Autodesk Fusion 360 part; units mm, degrees
(part 4 of 6)
sketch "b back lines" plane through (0, 0, 0) normal (0, 0, 1) x (1, 0, 0) in component "b back component"
  line L0 (155.185, 125.185) -> (161.93, 125.185)
  line L1 (161.93, 125.185) -> (161.93, 122.01)
  line L2 (161.93, 122.01) -> (172.09, 122.01)
  line L3 (172.09, 122.01) -> (172.09, 125.185)
  line L4 (172.09, 125.185) -> (181.93, 125.185)
  line L5 (181.93, 125.185) -> (181.93, 122.01)
  line L6 (181.93, 122.01) -> (192.09, 122.01)
  line L7 (192.09, 122.01) -> (192.09, 125.185)
  line L8 (192.09, 125.185) -> (201.93, 125.185)
  line L9 (201.93, 125.185) -> (201.93, 122.01)
  line L10 (201.93, 122.01) -> (212.09, 122.01)
  line L11 (212.09, 122.01) -> (212.09, 125.185)
  line L12 (212.09, 125.185) -> (221.93, 125.185)
  line L13 (221.93, 125.185) -> (221.93, 122.01)
  line L14 (221.93, 122.01) -> (232.09, 122.01)
  line L15 (232.09, 122.01) -> (232.09, 125.185)
  line L16 (232.09, 125.185) -> (241.93, 125.185)
  line L17 (241.93, 125.185) -> (241.93, 122.01)
  line L18 (241.93, 122.01) -> (252.09, 122.01)
  line L19 (252.09, 122.01) -> (252.09, 125.185)
  line L20 (252.09, 125.185) -> (261.93, 125.185)
  line L21 (261.93, 125.185) -> (261.93, 122.01)
  line L22 (261.93, 122.01) -> (272.09, 122.01)
  line L23 (272.09, 122.01) -> (272.09, 125.185)
  line L24 (272.09, 125.185) -> (281.93, 125.185)
  line L25 (281.93, 125.185) -> (281.93, 122.01)
  line L26 (281.93, 122.01) -> (292.09, 122.01)
  line L27 (292.09, 122.01) -> (292.09, 125.185)
  line L28 (292.09, 125.185) -> (298.835, 125.185)
  line L29 (298.835, 125.185) -> (298.835, 139.43)
  line L30 (298.835, 139.43) -> (302.01, 139.43)
  line L31 (302.01, 139.43) -> (302.01, 149.59)
  line L32 (302.01, 149.59) -> (298.835, 149.59)
  line L33 (298.835, 149.59) -> (298.835, 159.43)
  line L34 (298.835, 159.43) -> (302.01, 159.43)
  line L35 (302.01, 159.43) -> (302.01, 169.59)
  line L36 (302.01, 169.59) -> (298.835, 169.59)
  line L37 (298.835, 169.59) -> (298.835, 183.835)
  line L38 (155.185, 183.835) -> (161.93, 183.835)
  line L39 (161.93, 183.835) -> (161.93, 187.01)
  line L40 (161.93, 187.01) -> (172.09, 187.01)
  line L41 (172.09, 187.01) -> (172.09, 183.835)
  line L42 (172.09, 183.835) -> (181.93, 183.835)
  line L43 (181.93, 183.835) -> (181.93, 187.01)
  line L44 (181.93, 187.01) -> (192.09, 187.01)
  line L45 (192.09, 187.01) -> (192.09, 183.835)
  line L46 (192.09, 183.835) -> (201.93, 183.835)
  line L47 (201.93, 183.835) -> (201.93, 187.01)
  line L48 (201.93, 187.01) -> (212.09, 187.01)
  line L49 (212.09, 187.01) -> (212.09, 183.835)
  line L50 (212.09, 183.835) -> (221.93, 183.835)
  line L51 (221.93, 183.835) -> (221.93, 187.01)
  line L52 (221.93, 187.01) -> (232.09, 187.01)
  line L53 (232.09, 187.01) -> (232.09, 183.835)
  line L54 (232.09, 183.835) -> (241.93, 183.835)
  line L55 (241.93, 183.835) -> (241.93, 187.01)
  line L56 (241.93, 187.01) -> (252.09, 187.01)
  line L57 (252.09, 187.01) -> (252.09, 183.835)
  line L58 (252.09, 183.835) -> (261.93, 183.835)
  line L59 (261.93, 183.835) -> (261.93, 187.01)
  line L60 (261.93, 187.01) -> (272.09, 187.01)
  line L61 (272.09, 187.01) -> (272.09, 183.835)
  line L62 (272.09, 183.835) -> (281.93, 183.835)
  line L63 (281.93, 183.835) -> (281.93, 187.01)
  line L64 (281.93, 187.01) -> (292.09, 187.01)
  line L65 (292.09, 187.01) -> (292.09, 183.835)
  line L66 (292.09, 183.835) -> (298.835, 183.835)
  line L67 (155.185, 125.185) -> (155.185, 139.43)
  line L68 (155.185, 139.43) -> (152.01, 139.43)
  line L69 (152.01, 139.43) -> (152.01, 149.59)
  line L70 (152.01, 149.59) -> (155.185, 149.59)
  line L71 (155.185, 149.59) -> (155.185, 159.43)
  line L72 (155.185, 159.43) -> (152.01, 159.43)
  line L73 (152.01, 159.43) -> (152.01, 169.59)
  line L74 (152.01, 169.59) -> (155.185, 169.59)
  line L75 (155.185, 169.59) -> (155.185, 183.835)
  dimension "d5610" = 6.745
  dimension "d5611" = 3.175
  dimension "d5612" = 10.16
  dimension "d5613" = 3.175
  dimension "d5614" = 9.84
  dimension "d5615" = 3.175
  dimension "d5616" = 10.16
  dimension "d5617" = 3.175
  dimension "d5618" = 9.84
  dimension "d5619" = 3.175
  dimension "d5620" = 10.16
  dimension "d5621" = 3.175
  dimension "d5622" = 9.84
  dimension "d5623" = 3.175
  dimension "d5624" = 10.16
  dimension "d5625" = 3.175
  dimension "d5626" = 9.84
  dimension "d5627" = 3.175
  dimension "d5628" = 10.16
  dimension "d5629" = 3.175
  dimension "d5630" = 9.84
  dimension "d5631" = 3.175
  dimension "d5632" = 10.16
  dimension "d5633" = 3.175
  dimension "d5634" = 9.84
  dimension "d5635" = 3.175
  dimension "d5636" = 10.16
  dimension "d5637" = 3.175
  dimension "d5638" = 6.745
  dimension "d5653" = 14.245
  dimension "d5654" = 3.175
  dimension "d5655" = 10.16
  dimension "d5656" = 3.175
  dimension "d5657" = 9.84
  dimension "d5658" = 3.175
  dimension "d5659" = 10.16
  dimension "d5660" = 3.175
  dimension "d5661" = 14.245
  dimension "d5666" = 6.745
  dimension "d5667" = 3.175
  dimension "d5668" = 10.16
  dimension "d5669" = 3.175
  dimension "d5670" = 9.84
  dimension "d5671" = 3.175
  dimension "d5672" = 10.16
  dimension "d5673" = 3.175
  dimension "d5674" = 9.84
  dimension "d5675" = 3.175
  dimension "d5676" = 10.16
  dimension "d5677" = 3.175
  dimension "d5678" = 9.84
  dimension "d5679" = 3.175
  dimension "d5680" = 10.16
  dimension "d5681" = 3.175
  dimension "d5682" = 9.84
  dimension "d5683" = 3.175
  dimension "d5684" = 10.16
  dimension "d5685" = 3.175
  dimension "d5686" = 9.84
  dimension "d5687" = 3.175
  dimension "d5688" = 10.16
  dimension "d5689" = 3.175
  dimension "d5690" = 9.84
  dimension "d5691" = 3.175
  dimension "d5692" = 10.16
  dimension "d5693" = 3.175
  dimension "d5694" = 6.745
  dimension "d5709" = 14.245
  dimension "d5710" = 3.175
  dimension "d5711" = 10.16
  dimension "d5712" = 3.175
  dimension "d5713" = 9.84
  dimension "d5714" = 3.175
  dimension "d5715" = 10.16
  dimension "d5716" = 3.175
  dimension "d5717" = 14.245
  constraint horizontal L0
  constraint vertical L1
  constraint horizontal L2
  constraint vertical L3
  constraint horizontal L4
  constraint vertical L5
  constraint horizontal L6
  constraint vertical L7
  constraint horizontal L8
  constraint vertical L9
  constraint horizontal L10
  constraint vertical L11
  constraint horizontal L12
  constraint vertical L13
  constraint horizontal L14
  constraint vertical L15
  constraint horizontal L16
  constraint vertical L17
  constraint horizontal L18
  constraint vertical L19
  constraint horizontal L20
  constraint vertical L21
  constraint horizontal L22
  constraint vertical L23
  constraint horizontal L24
  constraint vertical L25
  constraint horizontal L26
  constraint vertical L27
  constraint horizontal L28
  constraint vertical L29
  constraint horizontal L30
  constraint vertical L31
  constraint horizontal L32
  constraint vertical L33
  constraint horizontal L34
  constraint vertical L35
  constraint horizontal L36
  constraint vertical L37
  constraint horizontal L38
  constraint vertical L39
  constraint horizontal L40
  constraint vertical L41
  constraint horizontal L42
  constraint vertical L43
  constraint horizontal L44
  constraint vertical L45
  constraint horizontal L46
  constraint vertical L47
  constraint horizontal L48
  constraint vertical L49
  constraint horizontal L50
  constraint vertical L51
  constraint horizontal L52
  constraint vertical L53
  constraint horizontal L54
  constraint vertical L55
  constraint horizontal L56
  constraint vertical L57
  constraint horizontal L58
  constraint vertical L59
  constraint horizontal L60
  constraint vertical L61
  constraint horizontal L62
  constraint vertical L63
  constraint horizontal L64
  constraint vertical L65
  constraint horizontal L66
  constraint vertical L67
  constraint horizontal L68
  constraint vertical L69
  constraint horizontal L70
  constraint vertical L71
  constraint horizontal L72
  constraint vertical L73
  constraint horizontal L74
  constraint vertical L75
  measures "d5610" distance of L0.start L0.end
  measures "d5611" distance of L0.end L1.end
  measures "d5612" distance of L1.end L2.end
  measures "d5613" distance of L2.end L3.end
  measures "d5614" distance of L3.end L4.end
  measures "d5615" distance of L4.end L5.end
  measures "d5616" distance of L5.end L6.end
  measures "d5617" distance of L6.end L7.end
  measures "d5618" distance of L7.end L8.end
  measures "d5619" distance of L8.end L9.end
  measures "d5620" distance of L9.end L10.end
  measures "d5621" distance of L10.end L11.end
  measures "d5622" distance of L11.end L12.end
  measures "d5623" distance of L12.end L13.end
  measures "d5624" distance of L13.end L14.end
  measures "d5625" distance of L14.end L15.end
  measures "d5626" distance of L15.end L16.end
  measures "d5627" distance of L16.end L17.end
  measures "d5628" distance of L17.end L18.end
  measures "d5629" distance of L18.end L19.end
  measures "d5630" distance of L19.end L20.end
  measures "d5631" distance of L20.end L21.end
  measures "d5632" distance of L21.end L22.end
  measures "d5633" distance of L22.end L23.end
  measures "d5634" distance of L23.end L24.end
  measures "d5635" distance of L24.end L25.end
  measures "d5636" distance of L25.end L26.end
  measures "d5637" distance of L26.end L27.end
  measures "d5638" distance of L27.end L28.end
  measures "d5653" distance of L28.end L29.end
  measures "d5654" distance of L29.end L30.end
  measures "d5655" distance of L30.end L31.end
  measures "d5656" distance of L31.end L32.end
  measures "d5657" distance of L32.end L33.end
  measures "d5658" distance of L33.end L34.end
  measures "d5659" distance of L34.end L35.end
  measures "d5660" distance of L35.end L36.end
  measures "d5661" distance of L36.end L37.end
  measures "d5666" distance of L38.start L38.end
  measures "d5667" distance of L38.end L39.end
  measures "d5668" distance of L39.end L40.end
  measures "d5669" distance of L40.end L41.end
  measures "d5670" distance of L41.end L42.end
  measures "d5671" distance of L42.end L43.end
  measures "d5672" distance of L43.end L44.end
  measures "d5673" distance of L44.end L45.end
  measures "d5674" distance of L45.end L46.end
  measures "d5675" distance of L46.end L47.end
  measures "d5676" distance of L47.end L48.end
  measures "d5677" distance of L48.end L49.end
  measures "d5678" distance of L49.end L50.end
  measures "d5679" distance of L50.end L51.end
  measures "d5680" distance of L51.end L52.end
  measures "d5681" distance of L52.end L53.end
  measures "d5682" distance of L53.end L54.end
  measures "d5683" distance of L54.end L55.end
  measures "d5684" distance of L55.end L56.end
  measures "d5685" distance of L56.end L57.end
  measures "d5686" distance of L57.end L58.end
  measures "d5687" distance of L58.end L59.end
  measures "d5688" distance of L59.end L60.end
  measures "d5689" distance of L60.end L61.end
  measures "d5690" distance of L61.end L62.end
  measures "d5691" distance of L62.end L63.end
  measures "d5692" distance of L63.end L64.end
  measures "d5693" distance of L64.end L65.end
  measures "d5694" distance of L37.end L65.end
  measures "d5709" distance of L0.start L67.end
  measures "d5710" distance of L67.end L68.end
  measures "d5711" distance of L68.end L69.end
  measures "d5712" distance of L69.end L70.end
  measures "d5713" distance of L70.end L71.end
  measures "d5714" distance of L71.end L72.end
  measures "d5715" distance of L72.end L73.end
  measures "d5716" distance of L73.end L74.end
  measures "d5717" distance of L38.start L74.end
sketch "b back circles" plane through (0, 0, 0) normal (0, 0, 1) x (1, 0, 0) in component "b back component"
  line L0 (152.01, 122.01) -> (302.01, 122.01)
  line L1 (302.01, 122.01) -> (302.01, 187.01)
  line L2 (302.01, 187.01) -> (152.01, 187.01)
  line L3 (152.01, 187.01) -> (152.01, 122.01)
  circle A0 centre (161.3154, 124.3744) radius 1.005
  circle A1 centre (172.7046, 124.3744) radius 1.005
  circle A2 centre (181.3154, 124.3744) radius 1.005
  circle A3 centre (192.7046, 124.3744) radius 1.005
  circle A4 centre (201.3154, 124.3744) radius 1.005
  circle A5 centre (212.7046, 124.3744) radius 1.005
  circle A6 centre (221.3154, 124.3744) radius 1.005
  circle A7 centre (232.7046, 124.3744) radius 1.005
  circle A8 centre (241.3154, 124.3744) radius 1.005
  circle A9 centre (252.7046, 124.3744) radius 1.005
  circle A10 centre (261.3154, 124.3744) radius 1.005
  circle A11 centre (272.7046, 124.3744) radius 1.005
  circle A12 centre (281.3154, 124.3744) radius 1.005
  circle A13 centre (292.7046, 124.3744) radius 1.005
  circle A14 centre (299.6456, 138.8154) radius 1.005
  circle A15 centre (299.6456, 150.2046) radius 1.005
  circle A16 centre (299.6456, 158.8154) radius 1.005
  circle A17 centre (299.6456, 170.2046) radius 1.005
  circle A18 centre (161.3154, 184.6456) radius 1.005
  circle A19 centre (172.7046, 184.6456) radius 1.005
  circle A20 centre (181.3154, 184.6456) radius 1.005
  circle A21 centre (192.7046, 184.6456) radius 1.005
  circle A22 centre (201.3154, 184.6456) radius 1.005
  circle A23 centre (212.7046, 184.6456) radius 1.005
  circle A24 centre (221.3154, 184.6456) radius 1.005
  circle A25 centre (232.7046, 184.6456) radius 1.005
  circle A26 centre (241.3154, 184.6456) radius 1.005
  circle A27 centre (252.7046, 184.6456) radius 1.005
  circle A28 centre (261.3154, 184.6456) radius 1.005
  circle A29 centre (272.7046, 184.6456) radius 1.005
  circle A30 centre (281.3154, 184.6456) radius 1.005
  circle A31 centre (292.7046, 184.6456) radius 1.005
  circle A32 centre (154.3744, 138.8154) radius 1.005
  circle A33 centre (154.3744, 150.2046) radius 1.005
  circle A34 centre (154.3744, 158.8154) radius 1.005
  circle A35 centre (154.3744, 170.2046) radius 1.005
  dimension "d5639" = 2.01
  dimension "d5640" = 2.01
  dimension "d5641" = 2.01
  dimension "d5642" = 2.01
  dimension "d5643" = 2.01
  dimension "d5644" = 2.01
  dimension "d5645" = 2.01
  dimension "d5646" = 2.01
  dimension "d5647" = 2.01
  dimension "d5648" = 2.01
  dimension "d5649" = 2.01
  dimension "d5650" = 2.01
  dimension "d5651" = 2.01
  dimension "d5652" = 2.01
  dimension "d5662" = 2.01
  dimension "d5663" = 2.01
  dimension "d5664" = 2.01
  dimension "d5665" = 2.01
  dimension "d5695" = 2.01
  dimension "d5696" = 2.01
  dimension "d5697" = 2.01
  dimension "d5698" = 2.01
  dimension "d5699" = 2.01
  dimension "d5700" = 2.01
  dimension "d5701" = 2.01
  dimension "d5702" = 2.01
  dimension "d5703" = 2.01
  dimension "d5704" = 2.01
  dimension "d5705" = 2.01
  dimension "d5706" = 2.01
  dimension "d5707" = 2.01
  dimension "d5708" = 2.01
  dimension "d5718" = 2.01
  dimension "d5719" = 2.01
  dimension "d5720" = 2.01
  dimension "d5721" = 2.01
  measures "d5639" diameter of A0
  measures "d5640" diameter of A1
  measures "d5641" diameter of A2
  measures "d5642" diameter of A3
  measures "d5643" diameter of A4
  measures "d5644" diameter of A5
  measures "d5645" diameter of A6
  measures "d5646" diameter of A7
  measures "d5647" diameter of A8
  measures "d5648" diameter of A9
  measures "d5649" diameter of A10
  measures "d5650" diameter of A11
  measures "d5651" diameter of A12
  measures "d5652" diameter of A13
  measures "d5662" diameter of A14
  measures "d5663" diameter of A15
  measures "d5664" diameter of A16
  measures "d5665" diameter of A17
  measures "d5695" diameter of A18
  measures "d5696" diameter of A19
  measures "d5697" diameter of A20
  measures "d5698" diameter of A21
  measures "d5699" diameter of A22
  measures "d5700" diameter of A23
  measures "d5701" diameter of A24
  measures "d5702" diameter of A25
  measures "d5703" diameter of A26
  measures "d5704" diameter of A27
  measures "d5705" diameter of A28
  measures "d5706" diameter of A29
  measures "d5707" diameter of A30
  measures "d5708" diameter of A31
  measures "d5718" diameter of A32
  measures "d5719" diameter of A33
  measures "d5720" diameter of A34
  measures "d5721" diameter of A35
extrude "b back lines body extrude" add sketch "b back lines" along normal blind 3.175 separate body makes body 8 in component "b back component"
extrude "b back circles extrude" add sketch "b back circles" along normal blind 3.175 separate body makes body 9 in component "b back component"
combine "b back lines final combine feature" operation intersect target body 8 tool bodies 9 in component "b back component"
sketch "b back  projection" plane through (0, 0, 0) normal (0, 0, 1) x (1, 0, 0) in component "b back component"
  arc A0 (298.835, 150.7987) -> (298.835, 149.6106) centre (299.6456, 150.2046) ccw
  arc A1 (298.835, 139.4094) -> (298.835, 138.2213) centre (299.6456, 138.8154) ccw
  arc A2 (300.4408, 159.43) -> (298.8505, 159.43) centre (299.6456, 158.8154) ccw
  arc A3 (292.09, 125.1695) -> (292.09, 123.5792) centre (292.7046, 124.3744) ccw
  arc A4 (298.835, 170.7987) -> (298.835, 169.6106) centre (299.6456, 170.2046) ccw
  arc A5 (281.9094, 125.185) -> (280.7213, 125.185) centre (281.3154, 124.3744) ccw
  arc A6 (292.09, 185.4408) -> (292.09, 183.8505) centre (292.7046, 184.6456) ccw
  arc A7 (272.09, 125.1695) -> (272.09, 123.5792) centre (272.7046, 124.3744) ccw
  arc A8 (280.7213, 183.835) -> (281.9094, 183.835) centre (281.3154, 184.6456) ccw
  arc A9 (261.9094, 125.185) -> (260.7213, 125.185) centre (261.3154, 124.3744) ccw
  arc A10 (272.09, 185.4408) -> (272.09, 183.8505) centre (272.7046, 184.6456) ccw
  arc A11 (252.09, 125.1695) -> (252.09, 123.5792) centre (252.7046, 124.3744) ccw
  arc A12 (260.7213, 183.835) -> (261.9094, 183.835) centre (261.3154, 184.6456) ccw
  arc A13 (241.9094, 125.185) -> (240.7213, 125.185) centre (241.3154, 124.3744) ccw
  arc A14 (252.09, 185.4408) -> (252.09, 183.8505) centre (252.7046, 184.6456) ccw
  arc A15 (232.09, 125.1695) -> (232.09, 123.5792) centre (232.7046, 124.3744) ccw
  arc A16 (240.7213, 183.835) -> (241.9094, 183.835) centre (241.3154, 184.6456) ccw
  arc A17 (221.9094, 125.185) -> (220.7213, 125.185) centre (221.3154, 124.3744) ccw
  arc A18 (232.09, 185.4408) -> (232.09, 183.8505) centre (232.7046, 184.6456) ccw
  arc A19 (212.09, 125.1695) -> (212.09, 123.5792) centre (212.7046, 124.3744) ccw
  arc A20 (220.7213, 183.835) -> (221.9094, 183.835) centre (221.3154, 184.6456) ccw
  arc A21 (201.9094, 125.185) -> (200.7213, 125.185) centre (201.3154, 124.3744) ccw
  arc A22 (212.09, 185.4408) -> (212.09, 183.8505) centre (212.7046, 184.6456) ccw
  arc A23 (192.09, 125.1695) -> (192.09, 123.5792) centre (192.7046, 124.3744) ccw
  arc A24 (200.7213, 183.835) -> (201.9094, 183.835) centre (201.3154, 184.6456) ccw
  arc A25 (181.9094, 125.185) -> (180.7213, 125.185) centre (181.3154, 124.3744) ccw
  arc A26 (192.09, 185.4408) -> (192.09, 183.8505) centre (192.7046, 184.6456) ccw
  arc A27 (172.09, 125.1695) -> (172.09, 123.5792) centre (172.7046, 124.3744) ccw
  arc A28 (180.7213, 183.835) -> (181.9094, 183.835) centre (181.3154, 184.6456) ccw
  arc A29 (161.9094, 125.185) -> (160.7213, 125.185) centre (161.3154, 124.3744) ccw
  arc A30 (172.09, 185.4408) -> (172.09, 183.8505) centre (172.7046, 184.6456) ccw
  arc A31 (155.1695, 139.43) -> (153.5792, 139.43) centre (154.3744, 138.8154) ccw
  arc A32 (160.7213, 183.835) -> (161.9094, 183.835) centre (161.3154, 184.6456) ccw
  arc A33 (155.185, 149.6106) -> (155.185, 150.7987) centre (154.3744, 150.2046) ccw
  arc A34 (155.1695, 159.43) -> (153.5792, 159.43) centre (154.3744, 158.8154) ccw
  arc A35 (153.5792, 169.59) -> (155.1695, 169.59) centre (154.3744, 170.2046) ccw
  arc A36 (281.93, 123.5792) -> (281.93, 125.1695) centre (281.3154, 124.3744) ccw
  arc A37 (293.2987, 125.185) -> (292.1106, 125.185) centre (292.7046, 124.3744) ccw
  arc A38 (273.2987, 125.185) -> (272.1106, 125.185) centre (272.7046, 124.3744) ccw
  arc A39 (193.2987, 125.185) -> (192.1106, 125.185) centre (192.7046, 124.3744) ccw
  arc A40 (173.2987, 125.185) -> (172.1106, 125.185) centre (172.7046, 124.3744) ccw
  arc A41 (213.2987, 125.185) -> (212.1106, 125.185) centre (212.7046, 124.3744) ccw
  arc A42 (261.93, 123.5792) -> (261.93, 125.1695) centre (261.3154, 124.3744) ccw
  arc A43 (221.93, 123.5792) -> (221.93, 125.1695) centre (221.3154, 124.3744) ccw
  arc A44 (253.2987, 125.185) -> (252.1106, 125.185) centre (252.7046, 124.3744) ccw
  arc A45 (161.93, 123.5792) -> (161.93, 125.1695) centre (161.3154, 124.3744) ccw
  arc A46 (181.93, 123.5792) -> (181.93, 125.1695) centre (181.3154, 124.3744) ccw
  arc A47 (241.93, 123.5792) -> (241.93, 125.1695) centre (241.3154, 124.3744) ccw
  arc A48 (233.2987, 125.185) -> (232.1106, 125.185) centre (232.7046, 124.3744) ccw
  arc A49 (201.93, 123.5792) -> (201.93, 125.1695) centre (201.3154, 124.3744) ccw
  arc A50 (155.185, 169.6106) -> (155.185, 170.7987) centre (154.3744, 170.2046) ccw
  arc A51 (155.185, 158.2213) -> (155.185, 159.4094) centre (154.3744, 158.8154) ccw
  arc A52 (153.5792, 149.59) -> (155.1695, 149.59) centre (154.3744, 150.2046) ccw
  arc A53 (155.185, 138.2213) -> (155.185, 139.4094) centre (154.3744, 138.8154) ccw
  arc A54 (292.1106, 183.835) -> (293.2987, 183.835) centre (292.7046, 184.6456) ccw
  arc A55 (281.93, 183.8505) -> (281.93, 185.4408) centre (281.3154, 184.6456) ccw
  arc A56 (272.1106, 183.835) -> (273.2987, 183.835) centre (272.7046, 184.6456) ccw
  arc A57 (261.93, 183.8505) -> (261.93, 185.4408) centre (261.3154, 184.6456) ccw
  arc A58 (252.1106, 183.835) -> (253.2987, 183.835) centre (252.7046, 184.6456) ccw
  arc A59 (241.93, 183.8505) -> (241.93, 185.4408) centre (241.3154, 184.6456) ccw
  arc A60 (232.1106, 183.835) -> (233.2987, 183.835) centre (232.7046, 184.6456) ccw
  arc A61 (221.93, 183.8505) -> (221.93, 185.4408) centre (221.3154, 184.6456) ccw
  arc A62 (212.1106, 183.835) -> (213.2987, 183.835) centre (212.7046, 184.6456) ccw
  arc A63 (201.93, 183.8505) -> (201.93, 185.4408) centre (201.3154, 184.6456) ccw
  arc A64 (192.1106, 183.835) -> (193.2987, 183.835) centre (192.7046, 184.6456) ccw
  arc A65 (181.93, 183.8505) -> (181.93, 185.4408) centre (181.3154, 184.6456) ccw
  arc A66 (172.1106, 183.835) -> (173.2987, 183.835) centre (172.7046, 184.6456) ccw
  arc A67 (161.93, 183.8505) -> (161.93, 185.4408) centre (161.3154, 184.6456) ccw
  arc A68 (298.8505, 169.59) -> (300.4408, 169.59) centre (299.6456, 170.2046) ccw
  arc A69 (298.835, 159.4094) -> (298.835, 158.2213) centre (299.6456, 158.8154) ccw
  arc A70 (298.8505, 149.59) -> (300.4408, 149.59) centre (299.6456, 150.2046) ccw
  arc A71 (300.4408, 139.43) -> (298.8505, 139.43) centre (299.6456, 138.8154) ccw
  line L0 (298.8505, 149.59) -> (298.835, 149.59)
  line L1 (302.01, 149.59) -> (300.4408, 149.59)
  line L2 (298.835, 139.43) -> (298.8505, 139.43)
  line L3 (300.4408, 139.43) -> (302.01, 139.43)
  line L4 (298.835, 125.185) -> (298.835, 138.2213)
  line L5 (298.835, 139.4094) -> (298.835, 139.43)
  line L6 (298.835, 159.4094) -> (298.835, 159.43)
  line L7 (298.835, 150.7987) -> (298.835, 158.2213)
  line L8 (298.835, 149.59) -> (298.835, 149.6106)
  line L9 (292.09, 125.185) -> (292.1106, 125.185)
  line L10 (293.2987, 125.185) -> (298.835, 125.185)
  line L11 (300.4408, 159.43) -> (302.01, 159.43)
  line L12 (298.835, 159.43) -> (298.8505, 159.43)
  line L13 (292.09, 122.01) -> (292.09, 123.5792)
  line L14 (292.09, 125.1695) -> (292.09, 125.185)
  line L15 (298.8505, 169.59) -> (298.835, 169.59)
  line L16 (302.01, 169.59) -> (300.4408, 169.59)
  line L17 (281.93, 125.185) -> (281.93, 125.1695)
  line L18 (281.93, 123.5792) -> (281.93, 122.01)
  line L19 (298.835, 170.7987) -> (298.835, 183.835)
  line L20 (298.835, 169.59) -> (298.835, 169.6106)
  line L21 (292.09, 183.835) -> (292.1106, 183.835)
  line L22 (293.2987, 183.835) -> (298.835, 183.835)
  line L23 (272.09, 125.185) -> (272.1106, 125.185)
  line L24 (273.2987, 125.185) -> (280.7213, 125.185)
  line L25 (281.9094, 125.185) -> (281.93, 125.185)
  line L26 (292.09, 187.01) -> (292.09, 185.4408)
  line L27 (292.09, 183.8505) -> (292.09, 183.835)
  line L28 (272.09, 122.01) -> (272.09, 123.5792)
  line L29 (272.09, 125.1695) -> (272.09, 125.185)
  line L30 (281.93, 183.835) -> (281.93, 183.8505)
  line L31 (281.93, 185.4408) -> (281.93, 187.01)
  line L32 (261.93, 125.185) -> (261.93, 125.1695)
  line L33 (261.93, 123.5792) -> (261.93, 122.01)
  line L34 (272.09, 183.835) -> (272.1106, 183.835)
  line L35 (273.2987, 183.835) -> (280.7213, 183.835)
  line L36 (281.9094, 183.835) -> (281.93, 183.835)
  line L37 (252.09, 125.185) -> (252.1106, 125.185)
  line L38 (253.2987, 125.185) -> (260.7213, 125.185)
  line L39 (261.9094, 125.185) -> (261.93, 125.185)
  line L40 (272.09, 187.01) -> (272.09, 185.4408)
  line L41 (272.09, 183.8505) -> (272.09, 183.835)
  line L42 (252.09, 122.01) -> (252.09, 123.5792)
  line L43 (252.09, 125.1695) -> (252.09, 125.185)
  line L44 (261.93, 183.835) -> (261.93, 183.8505)
  line L45 (261.93, 185.4408) -> (261.93, 187.01)
  line L46 (241.93, 125.185) -> (241.93, 125.1695)
  line L47 (241.93, 123.5792) -> (241.93, 122.01)
  line L48 (252.09, 183.835) -> (252.1106, 183.835)
  line L49 (253.2987, 183.835) -> (260.7213, 183.835)
  line L50 (261.9094, 183.835) -> (261.93, 183.835)
  line L51 (232.09, 125.185) -> (232.1106, 125.185)
  line L52 (233.2987, 125.185) -> (240.7213, 125.185)
  line L53 (241.9094, 125.185) -> (241.93, 125.185)
  line L54 (252.09, 187.01) -> (252.09, 185.4408)
  line L55 (252.09, 183.8505) -> (252.09, 183.835)
  line L56 (232.09, 122.01) -> (232.09, 123.5792)
  line L57 (232.09, 125.1695) -> (232.09, 125.185)
  line L58 (241.93, 183.835) -> (241.93, 183.8505)
  line L59 (241.93, 185.4408) -> (241.93, 187.01)
  line L60 (221.93, 125.185) -> (221.93, 125.1695)
  line L61 (221.93, 123.5792) -> (221.93, 122.01)
  line L62 (232.09, 183.835) -> (232.1106, 183.835)
  line L63 (233.2987, 183.835) -> (240.7213, 183.835)
  line L64 (241.9094, 183.835) -> (241.93, 183.835)
  line L65 (212.09, 125.185) -> (212.1106, 125.185)
  line L66 (213.2987, 125.185) -> (220.7213, 125.185)
  line L67 (221.9094, 125.185) -> (221.93, 125.185)
  line L68 (232.09, 187.01) -> (232.09, 185.4408)
  line L69 (232.09, 183.8505) -> (232.09, 183.835)
  line L70 (212.09, 122.01) -> (212.09, 123.5792)
  line L71 (212.09, 125.1695) -> (212.09, 125.185)
  line L72 (221.93, 183.835) -> (221.93, 183.8505)
  line L73 (221.93, 185.4408) -> (221.93, 187.01)
  line L74 (201.93, 125.185) -> (201.93, 125.1695)
  line L75 (201.93, 123.5792) -> (201.93, 122.01)
  line L76 (212.09, 183.835) -> (212.1106, 183.835)
  line L77 (213.2987, 183.835) -> (220.7213, 183.835)
  line L78 (221.9094, 183.835) -> (221.93, 183.835)
  line L79 (192.09, 125.185) -> (192.1106, 125.185)
  line L80 (193.2987, 125.185) -> (200.7213, 125.185)
  line L81 (201.9094, 125.185) -> (201.93, 125.185)
  line L82 (212.09, 187.01) -> (212.09, 185.4408)
  line L83 (212.09, 183.8505) -> (212.09, 183.835)
  line L84 (192.09, 122.01) -> (192.09, 123.5792)
  line L85 (192.09, 125.1695) -> (192.09, 125.185)
  line L86 (201.93, 183.835) -> (201.93, 183.8505)
  line L87 (201.93, 185.4408) -> (201.93, 187.01)
  line L88 (181.93, 125.185) -> (181.93, 125.1695)
  line L89 (181.93, 123.5792) -> (181.93, 122.01)
  line L90 (192.09, 183.835) -> (192.1106, 183.835)
  line L91 (193.2987, 183.835) -> (200.7213, 183.835)
  line L92 (201.9094, 183.835) -> (201.93, 183.835)
  line L93 (172.09, 125.185) -> (172.1106, 125.185)
  line L94 (173.2987, 125.185) -> (180.7213, 125.185)
  line L95 (181.9094, 125.185) -> (181.93, 125.185)
  line L96 (192.09, 187.01) -> (192.09, 185.4408)
  line L97 (192.09, 183.8505) -> (192.09, 183.835)
  line L98 (172.09, 122.01) -> (172.09, 123.5792)
  line L99 (172.09, 125.1695) -> (172.09, 125.185)
  line L100 (181.93, 183.835) -> (181.93, 183.8505)
  line L101 (181.93, 185.4408) -> (181.93, 187.01)
  line L102 (161.93, 125.185) -> (161.93, 125.1695)
  line L103 (161.93, 123.5792) -> (161.93, 122.01)
  line L104 (155.185, 125.185) -> (160.7213, 125.185)
  line L105 (161.9094, 125.185) -> (161.93, 125.185)
  line L106 (172.09, 183.835) -> (172.1106, 183.835)
  line L107 (173.2987, 183.835) -> (180.7213, 183.835)
  line L108 (181.9094, 183.835) -> (181.93, 183.835)
  line L109 (155.185, 139.4094) -> (155.185, 139.43)
  line L110 (155.185, 125.185) -> (155.185, 138.2213)
  line L111 (172.09, 187.01) -> (172.09, 185.4408)
  line L112 (172.09, 183.8505) -> (172.09, 183.835)
  line L113 (153.5792, 139.43) -> (152.01, 139.43)
  line L114 (155.185, 139.43) -> (155.1695, 139.43)
  line L115 (161.93, 183.835) -> (161.93, 183.8505)
  line L116 (161.93, 185.4408) -> (161.93, 187.01)
  line L117 (155.1695, 149.59) -> (155.185, 149.59)
  line L118 (152.01, 149.59) -> (153.5792, 149.59)
  line L119 (155.185, 183.835) -> (160.7213, 183.835)
  line L120 (161.9094, 183.835) -> (161.93, 183.835)
  line L121 (155.185, 159.4094) -> (155.185, 159.43)
  line L122 (155.185, 150.7987) -> (155.185, 158.2213)
  line L123 (155.185, 149.59) -> (155.185, 149.6106)
  line L124 (155.185, 169.59) -> (155.185, 169.6106)
  line L125 (155.185, 170.7987) -> (155.185, 183.835)
  line L126 (153.5792, 159.43) -> (152.01, 159.43)
  line L127 (155.185, 159.43) -> (155.1695, 159.43)
  line L128 (152.01, 169.59) -> (153.5792, 169.59)
  line L129 (155.1695, 169.59) -> (155.185, 169.59)
  line L130 (152.01, 139.43) -> (152.01, 149.59)
  line L131 (152.01, 159.43) -> (152.01, 169.59)
  line L132 (161.93, 187.01) -> (172.09, 187.01)
  line L133 (181.93, 187.01) -> (192.09, 187.01)
  line L134 (201.93, 187.01) -> (212.09, 187.01)
  line L135 (221.93, 187.01) -> (232.09, 187.01)
  line L136 (241.93, 187.01) -> (252.09, 187.01)
  line L137 (261.93, 187.01) -> (272.09, 187.01)
  line L138 (281.93, 187.01) -> (292.09, 187.01)
  line L139 (302.01, 159.43) -> (302.01, 169.59)
  line L140 (302.01, 139.43) -> (302.01, 149.59)
  line L141 (281.93, 122.01) -> (292.09, 122.01)
  line L142 (261.93, 122.01) -> (272.09, 122.01)
  line L143 (241.93, 122.01) -> (252.09, 122.01)
  line L144 (221.93, 122.01) -> (232.09, 122.01)
  line L145 (201.93, 122.01) -> (212.09, 122.01)
  line L146 (181.93, 122.01) -> (192.09, 122.01)
  line L147 (161.93, 122.01) -> (172.09, 122.01)
sketch "b left lines" plane through (0, 0, 0) normal (0, 0, 1) x (1, 0, 0) in component "b left component"
  line L0 (0, 192.195) -> (14.92, 192.195)
  line L1 (14.92, 192.195) -> (14.92, 189.02)
  line L2 (14.92, 189.02) -> (25.08, 189.02)
  line L3 (25.08, 189.02) -> (25.08, 192.195)
  line L4 (25.08, 192.195) -> (34.92, 192.195)
  line L5 (34.92, 192.195) -> (34.92, 189.02)
  line L6 (34.92, 189.02) -> (45.08, 189.02)
  line L7 (45.08, 189.02) -> (45.08, 192.195)
  line L8 (45.08, 192.195) -> (54.92, 192.195)
  line L9 (54.92, 192.195) -> (54.92, 189.02)
  line L10 (54.92, 189.02) -> (65.08, 189.02)
  line L11 (65.08, 189.02) -> (65.08, 192.195)
  line L12 (65.08, 192.195) -> (74.92, 192.195)
  line L13 (74.92, 192.195) -> (74.92, 189.02)
  line L14 (74.92, 189.02) -> (85.08, 189.02)
  line L15 (85.08, 189.02) -> (85.08, 192.195)
  line L16 (85.08, 192.195) -> (94.92, 192.195)
  line L17 (94.92, 192.195) -> (94.92, 189.02)
  line L18 (94.92, 189.02) -> (105.08, 189.02)
  line L19 (105.08, 189.02) -> (105.08, 192.195)
  line L20 (105.08, 192.195) -> (120, 192.195)
  line L21 (120, 192.195) -> (120, 206.6)
  line L22 (120, 206.6) -> (116.825, 206.6)
  line L23 (116.825, 206.6) -> (116.825, 216.44)
  line L24 (116.825, 216.44) -> (120, 216.44)
  line L25 (120, 216.44) -> (120, 226.6)
  line L26 (120, 226.6) -> (116.825, 226.6)
  line L27 (116.825, 226.6) -> (116.825, 236.44)
  line L28 (116.825, 236.44) -> (120, 236.44)
  line L29 (120, 236.44) -> (120, 250.845)
  line L30 (0, 250.845) -> (14.92, 250.845)
  line L31 (14.92, 250.845) -> (14.92, 254.02)
  line L32 (14.92, 254.02) -> (25.08, 254.02)
  line L33 (25.08, 254.02) -> (25.08, 250.845)
  line L34 (25.08, 250.845) -> (34.92, 250.845)
  line L35 (34.92, 250.845) -> (34.92, 254.02)
  line L36 (34.92, 254.02) -> (45.08, 254.02)
  line L37 (45.08, 254.02) -> (45.08, 250.845)
  line L38 (45.08, 250.845) -> (54.92, 250.845)
  line L39 (54.92, 250.845) -> (54.92, 254.02)
  line L40 (54.92, 254.02) -> (65.08, 254.02)
  line L41 (65.08, 254.02) -> (65.08, 250.845)
  line L42 (65.08, 250.845) -> (74.92, 250.845)
  line L43 (74.92, 250.845) -> (74.92, 254.02)
  line L44 (74.92, 254.02) -> (85.08, 254.02)
  line L45 (85.08, 254.02) -> (85.08, 250.845)
  line L46 (85.08, 250.845) -> (94.92, 250.845)
  line L47 (94.92, 250.845) -> (94.92, 254.02)
  line L48 (94.92, 254.02) -> (105.08, 254.02)
  line L49 (105.08, 254.02) -> (105.08, 250.845)
  line L50 (105.08, 250.845) -> (120, 250.845)
  line L51 (0, 192.195) -> (0, 206.6)
  line L52 (0, 206.6) -> (3.175, 206.6)
  line L53 (3.175, 206.6) -> (3.175, 216.44)
  line L54 (3.175, 216.44) -> (0, 216.44)
  line L55 (0, 216.44) -> (0, 226.6)
  line L56 (0, 226.6) -> (3.175, 226.6)
  line L57 (3.175, 226.6) -> (3.175, 236.44)
  line L58 (3.175, 236.44) -> (0, 236.44)
  line L59 (0, 236.44) -> (0, 250.845)
  dimension "d5726" = 14.92
  dimension "d5727" = 3.175
  dimension "d5728" = 10.16
  dimension "d5729" = 3.175
  dimension "d5730" = 9.84
  dimension "d5731" = 3.175
  dimension "d5732" = 10.16
  dimension "d5733" = 3.175
  dimension "d5734" = 9.84
  dimension "d5735" = 3.175
  dimension "d5736" = 10.16
  dimension "d5737" = 3.175
  dimension "d5738" = 9.84
  dimension "d5739" = 3.175
  dimension "d5740" = 10.16
  dimension "d5741" = 3.175
  dimension "d5742" = 9.84
  dimension "d5743" = 3.175
  dimension "d5744" = 10.16
  dimension "d5745" = 3.175
  dimension "d5746" = 14.92
  dimension "d5757" = 14.405
  dimension "d5758" = 3.175
  dimension "d5759" = 9.84
  dimension "d5760" = 3.175
  dimension "d5761" = 10.16
  dimension "d5762" = 3.175
  dimension "d5763" = 9.84
  dimension "d5764" = 3.175
  dimension "d5765" = 14.405
  dimension "d5770" = 14.92
  dimension "d5771" = 3.175
  dimension "d5772" = 10.16
  dimension "d5773" = 3.175
  dimension "d5774" = 9.84
  dimension "d5775" = 3.175
  dimension "d5776" = 10.16
  dimension "d5777" = 3.175
  dimension "d5778" = 9.84
  dimension "d5779" = 3.175
  dimension "d5780" = 10.16
  dimension "d5781" = 3.175
  dimension "d5782" = 9.84
  dimension "d5783" = 3.175
  dimension "d5784" = 10.16
  dimension "d5785" = 3.175
  dimension "d5786" = 9.84
  dimension "d5787" = 3.175
  dimension "d5788" = 10.16
  dimension "d5789" = 3.175
  dimension "d5790" = 14.92
  dimension "d5801" = 14.405
  dimension "d5802" = 3.175
  dimension "d5803" = 9.84
  dimension "d5804" = 3.175
  dimension "d5805" = 10.16
  dimension "d5806" = 3.175
  dimension "d5807" = 9.84
  dimension "d5808" = 3.175
  dimension "d5809" = 14.405
  constraint horizontal L0
  constraint vertical L1
  constraint horizontal L2
  constraint vertical L3
  constraint horizontal L4
  constraint vertical L5
  constraint horizontal L6
  constraint vertical L7
  constraint horizontal L8
  constraint vertical L9
  constraint horizontal L10
  constraint vertical L11
  constraint horizontal L12
  constraint vertical L13
  constraint horizontal L14
  constraint vertical L15
  constraint horizontal L16
  constraint vertical L17
  constraint horizontal L18
  constraint vertical L19
  constraint horizontal L20
  constraint vertical L21
  constraint horizontal L22
  constraint vertical L23
  constraint horizontal L24
  constraint vertical L25
  constraint horizontal L26
  constraint vertical L27
  constraint horizontal L28
  constraint vertical L29
  constraint horizontal L30
  constraint vertical L31
  constraint horizontal L32
  constraint vertical L33
  constraint horizontal L34
  constraint vertical L35
  constraint horizontal L36
  constraint vertical L37
  constraint horizontal L38
  constraint vertical L39
  constraint horizontal L40
  constraint vertical L41
  constraint horizontal L42
  constraint vertical L43
  constraint horizontal L44
  constraint vertical L45
  constraint horizontal L46
  constraint vertical L47
  constraint horizontal L48
  constraint vertical L49
  constraint horizontal L50
  constraint vertical L51
  constraint horizontal L52
  constraint vertical L53
  constraint horizontal L54
  constraint vertical L55
  constraint horizontal L56
  constraint vertical L57
  constraint horizontal L58
  constraint vertical L59
  measures "d5726" distance of L0.start L0.end
  measures "d5727" distance of L0.end L1.end
  measures "d5728" distance of L1.end L2.end
  measures "d5729" distance of L2.end L3.end
  measures "d5730" distance of L3.end L4.end
  measures "d5731" distance of L4.end L5.end
  measures "d5732" distance of L5.end L6.end
  measures "d5733" distance of L6.end L7.end
  measures "d5734" distance of L7.end L8.end
  measures "d5735" distance of L8.end L9.end
  measures "d5736" distance of L9.end L10.end
  measures "d5737" distance of L10.end L11.end
  measures "d5738" distance of L11.end L12.end
  measures "d5739" distance of L12.end L13.end
  measures "d5740" distance of L13.end L14.end
  measures "d5741" distance of L14.end L15.end
  measures "d5742" distance of L15.end L16.end
  measures "d5743" distance of L16.end L17.end
  measures "d5744" distance of L17.end L18.end
  measures "d5745" distance of L18.end L19.end
  measures "d5746" distance of L19.end L20.end
  measures "d5757" distance of L20.end L21.end
  measures "d5758" distance of L21.end L22.end
  measures "d5759" distance of L22.end L23.end
  measures "d5760" distance of L23.end L24.end
  measures "d5761" distance of L24.end L25.end
  measures "d5762" distance of L25.end L26.end
  measures "d5763" distance of L26.end L27.end
  measures "d5764" distance of L27.end L28.end
  measures "d5765" distance of L28.end L29.end
  measures "d5770" distance of L30.start L30.end
  measures "d5771" distance of L30.end L31.end
  measures "d5772" distance of L31.end L32.end
  measures "d5773" distance of L32.end L33.end
  measures "d5774" distance of L33.end L34.end
  measures "d5775" distance of L34.end L35.end
  measures "d5776" distance of L35.end L36.end
  measures "d5777" distance of L36.end L37.end
  measures "d5778" distance of L37.end L38.end
  measures "d5779" distance of L38.end L39.end
  measures "d5780" distance of L39.end L40.end
  measures "d5781" distance of L40.end L41.end
  measures "d5782" distance of L41.end L42.end
  measures "d5783" distance of L42.end L43.end
  measures "d5784" distance of L43.end L44.end
  measures "d5785" distance of L44.end L45.end
  measures "d5786" distance of L45.end L46.end
  measures "d5787" distance of L46.end L47.end
  measures "d5788" distance of L47.end L48.end
  measures "d5789" distance of L48.end L49.end
  measures "d5790" distance of L29.end L49.end
  measures "d5801" distance of L0.start L51.end
  measures "d5802" distance of L51.end L52.end
  measures "d5803" distance of L52.end L53.end
  measures "d5804" distance of L53.end L54.end
  measures "d5805" distance of L54.end L55.end
  measures "d5806" distance of L55.end L56.end
  measures "d5807" distance of L56.end L57.end
  measures "d5808" distance of L57.end L58.end
  measures "d5809" distance of L30.start L58.end
sketch "b left circles" plane through (0, 0, 0) normal (0, 0, 1) x (1, 0, 0) in component "b left component"
  line L0 (0, 189.02) -> (120, 189.02)
  line L1 (120, 189.02) -> (120, 254.02)
  line L2 (120, 254.02) -> (0, 254.02)
  line L3 (0, 254.02) -> (0, 189.02)
  circle A0 centre (14.3054, 191.3844) radius 1.005
  circle A1 centre (25.6946, 191.3844) radius 1.005
  circle A2 centre (34.3054, 191.3844) radius 1.005
  circle A3 centre (45.6946, 191.3844) radius 1.005
  circle A4 centre (54.3054, 191.3844) radius 1.005
  circle A5 centre (65.6946, 191.3844) radius 1.005
  circle A6 centre (74.3054, 191.3844) radius 1.005
  circle A7 centre (85.6946, 191.3844) radius 1.005
  circle A8 centre (94.3054, 191.3844) radius 1.005
  circle A9 centre (105.6946, 191.3844) radius 1.005
  circle A10 centre (117.6356, 207.2146) radius 1.005
  circle A11 centre (117.6356, 215.8254) radius 1.005
  circle A12 centre (117.6356, 227.2146) radius 1.005
  circle A13 centre (117.6356, 235.8254) radius 1.005
  circle A14 centre (14.3054, 251.6556) radius 1.005
  circle A15 centre (25.6946, 251.6556) radius 1.005
  circle A16 centre (34.3054, 251.6556) radius 1.005
  circle A17 centre (45.6946, 251.6556) radius 1.005
  circle A18 centre (54.3054, 251.6556) radius 1.005
  circle A19 centre (65.6946, 251.6556) radius 1.005
  circle A20 centre (74.3054, 251.6556) radius 1.005
  circle A21 centre (85.6946, 251.6556) radius 1.005
  circle A22 centre (94.3054, 251.6556) radius 1.005
  circle A23 centre (105.6946, 251.6556) radius 1.005
  circle A24 centre (2.3644, 207.2146) radius 1.005
  circle A25 centre (2.3644, 215.8254) radius 1.005
  circle A26 centre (2.3644, 227.2146) radius 1.005
  circle A27 centre (2.3644, 235.8254) radius 1.005
  dimension "d5747" = 2.01
  dimension "d5748" = 2.01
  dimension "d5749" = 2.01
  dimension "d5750" = 2.01
  dimension "d5751" = 2.01
  dimension "d5752" = 2.01
  dimension "d5753" = 2.01
  dimension "d5754" = 2.01
  dimension "d5755" = 2.01
  dimension "d5756" = 2.01
  dimension "d5766" = 2.01
  dimension "d5767" = 2.01
  dimension "d5768" = 2.01
  dimension "d5769" = 2.01
  dimension "d5791" = 2.01
  dimension "d5792" = 2.01
  dimension "d5793" = 2.01
  dimension "d5794" = 2.01
  dimension "d5795" = 2.01
  dimension "d5796" = 2.01
  dimension "d5797" = 2.01
  dimension "d5798" = 2.01
  dimension "d5799" = 2.01
  dimension "d5800" = 2.01
  dimension "d5810" = 2.01
  dimension "d5811" = 2.01
  dimension "d5812" = 2.01
  dimension "d5813" = 2.01
  measures "d5747" diameter of A0
  measures "d5748" diameter of A1
  measures "d5749" diameter of A2
  measures "d5750" diameter of A3
  measures "d5751" diameter of A4
  measures "d5752" diameter of A5
  measures "d5753" diameter of A6
  measures "d5754" diameter of A7
  measures "d5755" diameter of A8
  measures "d5756" diameter of A9
  measures "d5766" diameter of A10
  measures "d5767" diameter of A11
  measures "d5768" diameter of A12
  measures "d5769" diameter of A13
  measures "d5791" diameter of A14
  measures "d5792" diameter of A15
  measures "d5793" diameter of A16
  measures "d5794" diameter of A17
  measures "d5795" diameter of A18
  measures "d5796" diameter of A19
  measures "d5797" diameter of A20
  measures "d5798" diameter of A21
  measures "d5799" diameter of A22
  measures "d5800" diameter of A23
  measures "d5810" diameter of A24
  measures "d5811" diameter of A25
  measures "d5812" diameter of A26
  measures "d5813" diameter of A27
extrude "b left lines body extrude" add sketch "b left lines" along normal blind 3.175 separate body makes body 10 in component "b left component"
extrude "b left circles extrude" add sketch "b left circles" along normal blind 3.175 separate body makes body 11 in component "b left component"
combine "b left lines final combine feature" operation intersect target body 10 tool bodies 11 in component "b left component"